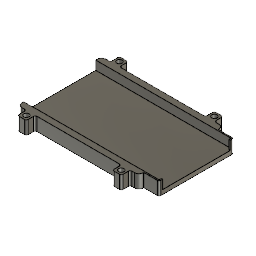
Assembled_v1 (Autodesk Fusion 360 archive; units mm, degrees)
design "fan_bottom_96"
Autodesk Fusion 360 part; units mm, degrees
(part 1 of 2)
sketch "Sketch1" plane through (0, 0, 0) normal (0, 0, 1) x (1, 0, 0)
  line L0 (-68.38, 47.37) -> (68.38, 47.37)
  line L1 (68.38, 47.37) -> (68.38, -47.37)
  line L2 (68.38, -47.37) -> (-68.38, -47.37)
  line L3 (-68.38, -47.37) -> (-68.38, 47.37)
  line L4 (-68.38, 47.37) -> (68.38, -47.37) construction
  line L5 (68.38, 47.37) -> (-68.38, -47.37) construction
  line L6 (-58.38, 57.37) -> (-48.38, 57.37)
  line L7 (-48.38, 57.37) -> (-48.38, 47.37)
  line L8 (-48.38, 47.37) -> (-58.38, 47.37)
  line L9 (-58.38, 47.37) -> (-58.38, 57.37)
  line L10 (48.38, 57.37) -> (58.38, 57.37)
  line L11 (58.38, 57.37) -> (58.38, 47.37)
  line L12 (58.38, 47.37) -> (48.38, 47.37)
  line L13 (48.38, 47.37) -> (48.38, 57.37)
  line L14 (48.38, -47.37) -> (58.38, -47.37)
  line L15 (58.38, -47.37) -> (58.38, -57.37)
  line L16 (58.38, -57.37) -> (48.38, -57.37)
  line L17 (48.38, -57.37) -> (48.38, -47.37)
  line L18 (-58.38, -47.37) -> (-48.38, -47.37)
  line L19 (-48.38, -47.37) -> (-48.38, -57.37)
  line L20 (-48.38, -57.37) -> (-58.38, -57.37)
  line L21 (-58.38, -57.37) -> (-58.38, -47.37)
  point P0 (-57.3369, -42.2056)
  point P1 (-53.88, -84.89)
  dimension "d1" = 136.76
  dimension "d2" = 94.74
  dimension "d3" = 10
  dimension "d4" = 10
  dimension "d5" = 10
  dimension "d6" = 10
  constraint perpendicular L0 L1
  constraint parallel L0 L2
  constraint parallel L1 L3
  constraint horizontal L0
  constraint horizontal L6
  constraint vertical L7
  constraint horizontal L8
  constraint vertical L9
  constraint coincident L0 L7.end
  constraint horizontal L10
  constraint vertical L11
  constraint horizontal L12
  constraint vertical L13
  constraint horizontal L14
  constraint vertical L15
  constraint horizontal L16
  constraint vertical L17
  constraint horizontal L18
  constraint vertical L19
  constraint horizontal L20
  constraint vertical L21
  measures "d1" distance of L1 L3
  measures "d2" distance of L0.start L2.end
  measures "d3" distance of L6.start L6.end
  measures "d4" distance of L6.start L8.end
  measures "d5" distance of L10.start L10.end
  measures "d6" distance of L10.start L12.end
extrude "Extrude1" add sketch "Sketch1" along normal blind 15
ref_plane "WorkPlane1" through (0, 0, 15) normal (0, 0, 1) x (1, 0, 0)
sketch "Sketch2" plane through (0, 0, 15) normal (0, 0, 1) x (1, 0, 0)
  line L0 (68.38, -40.5) -> (-68.38, -40.5)
  line L1 (-68.38, -40.5) -> (-68.38, 40.5)
  line L2 (-68.38, 40.5) -> (68.38, 40.5)
  line L3 (68.38, 40.5) -> (68.38, -40.5)
  line L4 (68.38, -40.5) -> (-68.38, 40.5) construction
  line L5 (-68.38, -40.5) -> (68.38, 40.5) construction
  dimension "d18" = 136.76
  dimension "d19" = 81
  constraint perpendicular L0 L1
  constraint parallel L0 L2
  constraint parallel L1 L3
  constraint horizontal L0
  constraint coincident L4 origin
  constraint coincident L5 origin
  measures "d18" distance of L1.end L2.end
  measures "d19" distance of L0.end L1.end
extrude "Extrude2" cut sketch "Sketch2" against normal blind 10
ref_plane "WorkPlane2" through (68.38, 0, 7.5) normal (1, 0, 0) x (0, 1, 0)
sketch "Sketch3" plane through (68.38, 0, 7.5) normal (1, 0, 0) x (0, 1, 0)
  line L0 (42, -7.5) -> (-42, -7.5)
  line L1 (-42, -7.5) -> (-42, 7.5)
  line L2 (-42, 7.5) -> (42, 7.5)
  line L3 (42, 7.5) -> (42, -7.5)
  line L4 (42, -7.5) -> (-42, 7.5) construction
  line L5 (-42, -7.5) -> (42, 7.5) construction
  dimension "d23" = 84
  dimension "d24" = 15
  constraint perpendicular L0 L1
  constraint parallel L0 L2
  constraint parallel L1 L3
  constraint horizontal L0
  constraint coincident L4 origin
  constraint coincident L5 origin
  measures "d23" distance of L1.end L2.end
  measures "d24" distance of L0.end L1.end
sketch "Sketch5" plane through (7.88, 0, 15) normal (0, 0, 1) x (1, 0, 0)
  circle A0 centre (-61.26, 52.37) radius 3
  circle A1 centre (45.5, 52.37) radius 3
  circle A2 centre (-61.26, -52.37) radius 3
  circle A3 centre (45.5, -52.37) radius 3
  dimension "d29" = 6
  dimension "d32" = 106.76
  dimension "d33" = -104.74
  measures "d29" diameter of A0
extrude "Extrude4" cut sketch "Sketch5" against normal blind 15
fillet "Fillet4" radius 5 4 edges at (68.38, 47.37, 7.5) (-68.38, 47.37, 7.5) (-68.38, -47.37, 7.5) (68.38, -47.37, 7.5)
ref_plane "WorkPlane7" through (68.38, 0, 7.5) normal (1, 0, 0) x (0, 1, 0)
fillet "Fillet5" radius 2 16 edges at (-58.38, -57.37, 7.5) (-48.38, -57.37, 7.5) (-48.38, -47.37, 7.5) (48.38, -57.37, 7.5) (58.38, -57.37, 7.5) (58.38, -47.37, 7.5) (58.38, 47.37, 7.5) (58.38, 57.37, 7.5) (48.38, 57.37, 7.5) (-48.38, 47.37, 7.5) (-48.38, 57.37, 7.5) (-58.38, 57.37, 7.5) (48.38, 47.37, 7.5) (-58.38, 47.37, 7.5) (-58.38, -47.37, 7.5) (48.38, -47.37, 7.5)
sketch "Sketch8" plane through (68.38, 0, 7.5) normal (1, 0, 0) x (0, 1, 0)
  line L0 (0, -7.5) -> (-42, -7.5)
  line L1 (-42, -7.5) -> (42, -7.5)
  line L2 (42, -7.5) -> (42, 7.5)
  line L3 (42, 7.5) -> (-42, 7.5)
  line L4 (-42, 7.5) -> (-42, -7.5)
  dimension "d52" = 42
  dimension "d53" = 84
  dimension "d54" = 15
  constraint horizontal L0
  constraint horizontal L1
  constraint vertical L2
  constraint horizontal L3
  constraint vertical L4
  measures "d52" distance of L0.start L0.end
  measures "d53" distance of L0.end L1.end
  measures "d54" distance of L0.end L3.end
extrude "Extrude6" add sketch "Sketch8" along normal blind 17.2
ref_plane "WorkPlane9" through (8.6, 0, 15) normal (0, 0, 1) x (1, 0, 0)
sketch "Sketch10" plane through (8.6, 0, 15) normal (0, 0, 1) x (1, 0, 0)
  line L0 (75.48, -40.5) -> (44.08, -40.5)
  line L1 (44.08, -40.5) -> (44.08, 40.5)
  line L2 (44.08, 40.5) -> (75.48, 40.5)
  line L3 (75.48, 40.5) -> (75.48, -40.5)
  line L4 (75.48, -40.5) -> (44.08, 40.5) construction
  line L5 (44.08, -40.5) -> (75.48, 40.5) construction
  point P0 (59.78, 0)
  dimension "d66" = 31.4
  dimension "d67" = 81
  constraint perpendicular L0 L1
  constraint parallel L0 L2
  constraint parallel L1 L3
  constraint horizontal L0
  constraint coincident L4 P0
  constraint coincident L5 P0
  measures "d66" distance of L1.end L2.end
  measures "d67" distance of L0.end L1.end
extrude "Extrude8" cut sketch "Sketch10" against normal blind 10
fillet "Fillet8" radius 2 2 edges at (85.58, 42, 7.5) (85.58, -42, 7.5)
ref_plane "WorkPlane11" through (85.58, 0, 7.5) normal (1, 0, 0) x (0, 0, -1)
sketch "Sketch12" plane through (85.58, 0, 7.5) normal (1, 0, 0) x (0, 1, 0)
  line L0 (38, -2.5) -> (-38, -2.5)
  line L1 (-38, -2.5) -> (-38, 17.5)
  line L2 (-38, 17.5) -> (38, 17.5)
  line L3 (38, 17.5) -> (38, -2.5)
  line L4 (38, -2.5) -> (-38, 17.5) construction
  line L5 (-38, -2.5) -> (38, 17.5) construction
  point P0 (0, 7.5)
  dimension "d73" = 76
  dimension "d74" = 20
  constraint perpendicular L0 L1
  constraint parallel L0 L2
  constraint parallel L1 L3
  constraint horizontal L0
  constraint coincident L4 P0
  constraint coincident L5 P0
  measures "d73" distance of L1.end L2.end
  measures "d74" distance of L0.end L1.end
extrude "Extrude9" cut sketch "Sketch12" against normal blind 1.5

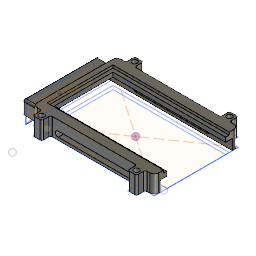
design "Mounting_plate_96_v2"
Autodesk Fusion 360 part; units mm, degrees
sketch "Sketch1" plane through (0, 0, 0) normal (0, 0, 1) x (1, 0, 0)
  line L0 (-68.38, 47.37) -> (68.38, 47.37)
  line L1 (68.38, 47.37) -> (68.38, -47.37)
  line L2 (68.38, -47.37) -> (-68.38, -47.37)
  line L3 (-68.38, -47.37) -> (-68.38, 47.37)
  line L4 (-68.38, 47.37) -> (68.38, -47.37) construction
  line L5 (68.38, 47.37) -> (-68.38, -47.37) construction
  line L6 (-58.38, 57.37) -> (-48.38, 57.37)
  line L7 (-48.38, 57.37) -> (-48.38, 47.37)
  line L8 (-48.38, 47.37) -> (-58.38, 47.37)
  line L9 (-58.38, 47.37) -> (-58.38, 57.37)
  line L10 (48.38, 57.37) -> (58.38, 57.37)
  line L11 (58.38, 57.37) -> (58.38, 47.37)
  line L12 (58.38, 47.37) -> (48.38, 47.37)
  line L13 (48.38, 47.37) -> (48.38, 57.37)
  line L14 (48.38, -47.37) -> (58.38, -47.37)
  line L15 (58.38, -47.37) -> (58.38, -57.37)
  line L16 (58.38, -57.37) -> (48.38, -57.37)
  line L17 (48.38, -57.37) -> (48.38, -47.37)
  line L18 (-58.38, -47.37) -> (-48.38, -47.37)
  line L19 (-48.38, -47.37) -> (-48.38, -57.37)
  line L20 (-48.38, -57.37) -> (-58.38, -57.37)
  line L21 (-58.38, -57.37) -> (-58.38, -47.37)
  line L22 (68.38, 47.37) -> (68.38, 37)
  line L23 (68.38, -47.37) -> (68.38, -36.63)
  line L24 (68.38, 37) -> (-62.58, 37)
  line L25 (-62.58, 37) -> (-62.58, -37)
  line L26 (-62.58, -37) -> (68.38, -37)
  line L27 (68.38, -37) -> (68.38, 37)
  line L28 (68.38, 37) -> (68.38, 33)
  line L29 (68.38, 33) -> (-58.58, 33)
  line L30 (-58.58, 33) -> (-58.58, -33)
  line L31 (-58.58, -33) -> (68.38, -33)
  line L32 (68.38, -33) -> (68.38, 33)
  point P0 (-57.3369, -42.2056)
  point P1 (-53.88, -84.89)
  dimension "d1" = 136.76
  dimension "d2" = 94.74
  dimension "d3" = 10
  dimension "d4" = 10
  dimension "d5" = 10
  dimension "d6" = 10
  dimension "d15" = 10.37
  dimension "d16" = 10.74
  dimension "d17" = 74
  dimension "d18" = 130.96
  dimension "d19" = 4
  dimension "d20" = 66
  dimension "d21" = 126.96
  constraint perpendicular L0 L1
  constraint parallel L0 L2
  constraint parallel L1 L3
  constraint horizontal L0
  constraint horizontal L6
  constraint vertical L7
  constraint horizontal L8
  constraint vertical L9
  constraint coincident L0 L7.end
  constraint horizontal L10
  constraint vertical L11
  constraint horizontal L12
  constraint vertical L13
  constraint horizontal L14
  constraint vertical L15
  constraint horizontal L16
  constraint vertical L17
  constraint horizontal L18
  constraint vertical L19
  constraint horizontal L20
  constraint vertical L21
  constraint perpendicular L0 L22
  constraint perpendicular L2 L23
  constraint horizontal L24
  constraint vertical L25
  constraint horizontal L26
  constraint vertical L27
  constraint perpendicular L24 L28
  constraint horizontal L29
  constraint vertical L30
  constraint horizontal L31
  constraint vertical L32
  measures "d1" distance of L1 L3
  measures "d2" distance of L0.start L2.end
  measures "d3" distance of L6.start L6.end
  measures "d4" distance of L6.start L8.end
  measures "d5" distance of L10.start L10.end
  measures "d6" distance of L10.start L12.end
  measures "d15" distance of L0.end L22.end
  measures "d16" distance of L1.end L23.end
  measures "d17" distance of L22.end L26.end
  measures "d18" distance of L22.end L24.end
  measures "d19" distance of L22.end L28.end
  measures "d20" distance of L28.end L31.end
  measures "d21" distance of L28.end L29.end
extrude "Extrude2" add sketch "Sketch1" along normal blind 20 contours L0 L1 L2 L3 L8 L12 L14 L18 L22 L23 L24 L25 L26 | L0 L6 L7 L8 L9 | L2 L18 L19 L20 L21 | L0 L10 L11 L12 L13 | L2 L14 L15 L16 L17 | L1 L23 L24 L25 L26 L27 L28 L29 L30 L31 makes body 1
ref_plane "WorkPlane2" through (0, 0, 20) normal (0, 0, 1) x (1, 0, 0)
sketch "Sketch4" plane through (0, 0, 20) normal (0, 0, 1) x (1, 0, 0)
  line L0 (68.38, 37) -> (-62.58, 37)
  line L1 (-62.58, 37) -> (-62.58, -37)
  line L2 (-62.58, -37) -> (68.38, -37)
  line L3 (68.38, -37) -> (68.38, 37)
  dimension "d30" = 130.96
  dimension "d31" = 74
  constraint horizontal L0
  constraint vertical L1
  constraint horizontal L2
  constraint vertical L3
  measures "d30" distance of L0.start L0.end
  measures "d31" distance of L0.start L2.end
extrude "Extrude3" cut sketch "Sketch4" against normal blind 3 bodies 1
ref_plane "WorkPlane3" through (0, 0, 20) normal (0, 0, 1) x (1, 0, 0)
sketch "Sketch5" plane through (0, 0, 20) normal (0, 0, 1) x (1, 0, 0)
  circle A0 centre (-53.38, 52.37) radius 3
  circle A1 centre (53.38, 52.37) radius 3
  circle A2 centre (-53.38, -52.37) radius 3
  circle A3 centre (53.38, -52.37) radius 3
  dimension "d35" = 6
  dimension "d38" = 106.76
  dimension "d39" = -104.74
  measures "d35" diameter of A0
extrude "Extrude4" cut sketch "Sketch5" against normal blind 20 bodies 1
ref_plane "WorkPlane5" through (68.38, 0, 0) normal (1, 0, 0) x (0, 1, 0)
ref_plane "WorkPlane6" through (68.38, 0, 0) normal (1, 0, 0) x (0, 1, 0)
sketch "Sketch7" plane through (68.38, 0, 0) normal (1, 0, 0) x (0, 1, 0)
  line L0 (40.5, 12) -> (-40.5, 12)
  line L1 (-40.5, 12) -> (-40.5, -12)
  line L2 (-40.5, -12) -> (40.5, -12)
  line L3 (40.5, -12) -> (40.5, 12)
  line L4 (40.5, 12) -> (-40.5, -12) construction
  line L5 (-40.5, 12) -> (40.5, -12) construction
  dimension "d45" = 81
  dimension "d46" = 24
  constraint perpendicular L0 L1
  constraint parallel L0 L2
  constraint parallel L1 L3
  constraint horizontal L0
  constraint coincident L4 origin
  constraint coincident L5 origin
  measures "d45" distance of L1.end L2.end
  measures "d46" distance of L0.end L1.end
extrude "Extrude5" cut sketch "Sketch7" against normal blind 136.76 bodies 1
fillet "Fillet1" radius 5 4 edges at (68.38, 47.37, 10) (-68.38, 47.37, 10) (-68.38, -47.37, 10) (68.38, -47.37, 10) on bodies 1
fillet "Fillet2" radius 2 16 edges at (-58.38, 57.37, 10) (-58.38, 47.37, 10) (-58.38, -47.37, 10) (-58.38, -57.37, 10) (-48.38, -57.37, 10) (-48.38, -47.37, 10) (58.38, -57.37, 10) (58.38, -47.37, 10) (48.38, -47.37, 10) (48.38, -57.37, 10) (58.38, 47.37, 10) (58.38, 57.37, 10) (48.38, 47.37, 10) (48.38, 57.37, 10) (-48.38, 47.37, 10) (-48.38, 57.37, 10) on bodies 1
ref_plane "WorkPlane7" through (0, -47.37, 10) normal (0, -1, 0) x (1, 0, 0)
delete_face "DeleteFace1" 1 faces at (15.46, -47.37, 6.6667) on bodies 1
ref_plane "WorkPlane9" through (0, -47.37, 10) normal (0, -1, 0) x (1, 0, 0)
sketch "Sketch10" plane through (0, -47.37, 10) normal (0, -1, 0) x (1, 0, 0)
  line L0 (0, -10) -> (0, -4)
  line L1 (40, -7) -> (-40, -7)
  line L2 (-40, -7) -> (-40, -1)
  line L3 (-40, -1) -> (40, -1)
  line L4 (40, -1) -> (40, -7)
  line L5 (40, -7) -> (-40, -1) construction
  line L6 (-40, -7) -> (40, -1) construction
  circle A0 centre (-40, -4) radius 3
  circle A1 centre (40, -4) radius 3
  point P0 (0, -4)
  dimension "d72" = 6
  dimension "d73" = 6
  dimension "d74" = 80
  dimension "d75" = 6
  dimension "d76" = 6
  constraint vertical L0
  constraint perpendicular L1 L2
  constraint parallel L1 L3
  constraint parallel L2 L4
  constraint horizontal L1
  constraint coincident L5 P0
  constraint coincident L6 P0
  constraint coincident P0 L0.end
  constraint midpoint L2 A0.centre
  constraint midpoint L4 A1.centre
  measures "d72" distance of L0.start P0
  measures "d73" distance of L1.end L2.end
  measures "d74" distance of L2.end L3.end
  measures "d75" diameter of A0
  measures "d76" diameter of A1
extrude "Extrude9" cut sketch "Sketch10" against normal blind 6.87 bodies 1
ref_plane "WorkPlane10" through (0, 47.37, 10) normal (0, 1, 0) x (-1, 0, 0)
sketch "Sketch11" plane through (0, 47.37, 10) normal (0, 1, 0) x (1, 0, 0)
  line L0 (0, 10) -> (0, 4)
  line L1 (-40, 7) -> (40, 7)
  line L2 (40, 7) -> (40, 1)
  line L3 (40, 1) -> (-40, 1)
  line L4 (-40, 1) -> (-40, 7)
  line L5 (-40, 7) -> (40, 1) construction
  line L6 (40, 7) -> (-40, 1) construction
  circle A0 centre (40, 4) radius 3
  circle A1 centre (-40, 4) radius 3
  point P0 (0, 4)
  dimension "d80" = 6
  dimension "d81" = 80
  dimension "d82" = 6
  dimension "d83" = 6
  dimension "d84" = 6
  constraint vertical L0
  constraint perpendicular L1 L2
  constraint parallel L1 L3
  constraint parallel L2 L4
  constraint horizontal L1
  constraint coincident L5 P0
  constraint coincident L6 P0
  constraint coincident P0 L0.end
  constraint midpoint L2 A0.centre
  constraint midpoint L4 A1.centre
  measures "d80" distance of L0.start P0
  measures "d81" distance of L2.end L3.end
  measures "d82" distance of L1.end L2.end
  measures "d83" diameter of A0
  measures "d84" diameter of A1
extrude "Extrude10" cut sketch "Sketch11" against normal blind 6.87 bodies 1
ref_plane "WorkPlane11" through (0, 0, 0) normal (0, 0, 1) x (1, 0, 0)
sketch "Sketch12" plane through (0, 0, 0) normal (0, 0, 1) x (1, 0, 0)
ref_plane "WorkPlane12" through (-68.38, 0, 10) normal (-1, 0, 0) x (0, -1, 0)
ref_plane "WorkPlane13" through (-68.38, 0, 10) normal (-1, 0, 0) x (0, -1, 0)
sketch "Sketch19" plane through (68.38, 0, 0) normal (1, 0, 0) x (0, 1, 0)
ref_plane "WorkPlane19" through (-68.38, 0, 10) normal (-1, 0, 0) x (0, -1, 0)
sketch "Sketch21" plane through (-68.38, 0, 10) normal (-1, 0, 0) x (0, 1, 0)
  line L0 (42, -2) -> (-42, -2)
  line L1 (42, -2) -> (-42, 22) construction
  line L2 (-42, -2) -> (42, 22) construction
  line L3 (42, -2) -> (-42, -2)
  line L4 (-42, -2) -> (-42, 10)
  line L5 (-42, 10) -> (42, 10)
  line L6 (42, 10) -> (42, -2)
  point P0 (0, 10)
  dimension "d112" = 84
  dimension "d113" = 24
  constraint horizontal L0
  constraint coincident L1 P0
  constraint coincident L2 P0
  constraint horizontal L3
  constraint vertical L4
  constraint horizontal L5
  constraint vertical L6
  measures "d112" distance of L1.end L2.end
  measures "d113" distance of L0.end L1.end
extrude "Extrude15" add sketch "Sketch21" along normal blind 17.2 separate body makes body 2
ref_plane "WorkPlane20" through (-68.32, 0, 0) normal (1, 0, 0) x (0, 1, 0)
sketch "Sketch22" plane through (-68.32, 0, 0) normal (1, 0, 0) x (0, 1, 0)
  line L0 (40.5, -12) -> (-40.5, -12)
  line L1 (-40.5, -12) -> (-40.5, 12)
  line L2 (-40.5, 12) -> (40.5, 12)
  line L3 (40.5, 12) -> (40.5, -12)
  line L4 (40.5, -12) -> (-40.5, 12) construction
  line L5 (-40.5, -12) -> (40.5, 12) construction
  dimension "d117" = 81
  dimension "d118" = 24
  constraint perpendicular L0 L1
  constraint parallel L0 L2
  constraint parallel L1 L3
  constraint horizontal L0
  constraint coincident L4 origin
  constraint coincident L5 origin
  measures "d117" distance of L1.end L2.end
  measures "d118" distance of L0.end L1.end
extrude "Extrude16" cut sketch "Sketch22" against normal blind 15.76 bodies 2
ref_plane "WorkPlane23" through (-76.98, 0, 12) normal (0, 0, 1) x (0, 1, 0)
sketch "Sketch25" plane through (-76.98, 0, 12) normal (0, 0, 1) x (1, 0, 0)
  line L0 (8.6, 42) -> (-8.6, 42)
  line L1 (-8.6, 42) -> (-8.6, -42)
  line L2 (-8.6, -42) -> (8.6, -42)
  line L3 (8.6, -42) -> (8.6, 42)
  dimension "d136" = 17.2
  dimension "d137" = 84
  constraint horizontal L0
  constraint vertical L1
  constraint horizontal L2
  constraint vertical L3
  measures "d136" distance of L0.start L0.end
  measures "d137" distance of L0.start L2.end
extrude "Extrude19" add sketch "Sketch25" along normal blind 3 bodies 1 2
fillet "Fillet5" radius 2 5 edges at (-76.98, 42, 15) (-85.58, 42, 7.5) (-85.58, 0, 15) (-76.98, -42, 15) (-85.58, -42, 7.5) on bodies 1
ref_plane "WorkPlane24" through (-85.58, 0, 6.5) normal (-1, 0, 0) x (0, -1, 0)
sketch "Sketch26" plane through (-85.58, 0, 6.5) normal (-1, 0, 0) x (0, 1, 0)
  line L0 (38, 18.5) -> (-38, 18.5)
  line L1 (-38, 18.5) -> (-38, -3.5)
  line L2 (-38, -3.5) -> (38, -3.5)
  line L3 (38, -3.5) -> (38, 18.5)
  line L4 (38, 18.5) -> (-38, -3.5) construction
  line L5 (-38, 18.5) -> (38, -3.5) construction
  point P0 (0, 7.5)
  dimension "d142" = 76
  dimension "d143" = 22
  constraint perpendicular L0 L1
  constraint parallel L0 L2
  constraint parallel L1 L3
  constraint horizontal L0
  constraint coincident L4 P0
  constraint coincident L5 P0
  measures "d142" distance of L1.end L2.end
  measures "d143" distance of L0.end L1.end
extrude "Extrude21" cut sketch "Sketch26" against normal blind 17.2 bodies 1
extrude "Extrude20" [rolled back] along distance -17.2 taper angle 0
fillet "Fillet3" [rolled back] radius 2
fillet "Fillet4" [rolled back] radius 2
ref_plane "WorkPlane21" through (-85.58, 0, 5) normal (-1, 0, 0) x (0, 0, 1)
ref_plane "WorkPlane22" through (-85.58, 0, 5) normal (-1, 0, 0) x (0, 0, 1)
sketch "Sketch24" plane through (-85.58, 0, 5) normal (-1, 0, 0) x (0, 1, 0)
  line L0 (-38, 11) -> (38, 11)
  line L1 (38, 11) -> (38, -3)
  line L2 (38, -3) -> (-38, -3)
  line L3 (-38, -3) -> (-38, 11)
  line L4 (-38, 11) -> (38, -3) construction
  line L5 (38, 11) -> (-38, -3) construction
  point P0 (0, 4)
  dimension "d131" = 76
  dimension "d132" = 14
  constraint perpendicular L0 L1
  constraint parallel L0 L2
  constraint parallel L1 L3
  constraint horizontal L0
  constraint coincident L4 P0
  constraint coincident L5 P0
  measures "d131" distance of L1.end L2.end
  measures "d132" distance of L0.end L1.end
extrude "Extrude18" [rolled back] along distance -1.5 taper angle 0

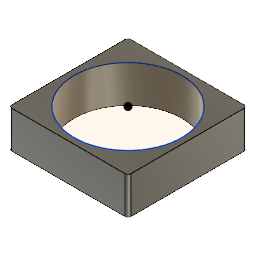
design "Fan"
Autodesk Fusion 360 part; units mm, degrees
sketch "Sketch1" plane through (0, 0, 0) normal (0, 0, 1) x (1, 0, 0)
  line L0 (40, -40) -> (-40, -40)
  line L1 (-40, -40) -> (-40, 40)
  line L2 (-40, 40) -> (40, 40)
  line L3 (40, 40) -> (40, -40)
  line L4 (40, -40) -> (-40, 40) construction
  line L5 (-40, -40) -> (40, 40) construction
  dimension "d1" = 80
  dimension "d2" = 80
  constraint perpendicular L0 L1
  constraint parallel L0 L2
  constraint parallel L1 L3
  constraint horizontal L0
  constraint coincident L4 origin
  constraint coincident L5 origin
  measures "d1" distance of L1.end L2.end
  measures "d2" distance of L0.end L1.end
extrude "Extrude1" add sketch "Sketch1" along normal blind 25
ref_plane "WorkPlane1" through (0, 0, 25) normal (0, 0, 1) x (1, 0, 0)
sketch "Sketch2" plane through (0, 0, 25) normal (0, 0, 1) x (1, 0, 0)
  circle A0 centre (0, 0) radius 36.0555
  constraint coincident A0.centre origin
extrude "Extrude3" cut sketch "Sketch2" against normal blind 25
fillet "Fillet1" radius 2 4 edges at (40, -40, 12.5) (40, 40, 12.5) (-40, 40, 12.5) (-40, -40, 12.5)

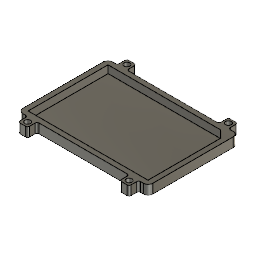
design "plate_lid_sketch"
Autodesk Fusion 360 part; units mm, degrees
sketch "Sketch1" plane through (0, 0, 0) normal (0, 0, 1) x (1, 0, 0)
  line L0 (68.38, -47.235) -> (-68.38, -47.235)
  line L1 (-68.38, -47.235) -> (-68.38, 47.235)
  line L2 (-68.38, 47.235) -> (68.38, 47.235)
  line L3 (68.38, 47.235) -> (68.38, -47.235)
  line L4 (68.38, -47.235) -> (-68.38, 47.235) construction
  line L5 (-68.38, -47.235) -> (68.38, 47.235) construction
  line L6 (-48.38, 47.235) -> (-58.38, 47.235)
  line L7 (-58.38, 47.235) -> (-58.38, 57.235)
  line L8 (-58.38, 57.235) -> (-48.38, 57.235)
  line L9 (-48.38, 57.235) -> (-48.38, 47.235)
  line L10 (-48.38, 47.235) -> (-58.38, 57.235) construction
  line L11 (-58.38, 47.235) -> (-48.38, 57.235) construction
  line L12 (48.38, 57.235) -> (58.38, 57.235)
  line L13 (48.38, 47.235) -> (48.38, 57.235)
  line L14 (58.38, 57.235) -> (58.38, 47.235)
  line L15 (58.38, 47.235) -> (48.38, 47.235)
  line L16 (48.38, -57.235) -> (48.38, -47.235)
  line L17 (48.38, -47.235) -> (58.38, -47.235)
  line L18 (58.38, -47.235) -> (58.38, -57.235)
  line L19 (48.38, -57.235) -> (58.38, -57.235)
  line L20 (-58.38, -57.235) -> (-58.38, -47.235)
  line L21 (-58.38, -47.235) -> (-48.38, -47.235)
  line L22 (-48.38, -47.235) -> (-48.38, -57.235)
  line L23 (-48.38, -57.235) -> (-58.38, -57.235)
  point P0 (-53.38, 52.235)
  dimension "d1" = 136.76
  dimension "d2" = 94.47
  dimension "d3" = 10
  dimension "d4" = 10
  dimension "d6" = 10
  dimension "d7" = 10
  constraint perpendicular L0 L1
  constraint parallel L0 L2
  constraint parallel L1 L3
  constraint horizontal L0
  constraint coincident L4 origin
  constraint coincident L5 origin
  constraint perpendicular L6 L7
  constraint parallel L6 L8
  constraint parallel L7 L9
  constraint horizontal L6
  constraint coincident L10 P0
  constraint coincident L11 P0
  constraint perpendicular L13 L15
  constraint parallel L12 L15
  constraint parallel L13 L14
  constraint horizontal L15
  constraint parallel L16 L18
  constraint perpendicular L18 L19
  constraint perpendicular L20 L23
  constraint parallel L21 L23
  constraint parallel L20 L22
  constraint horizontal L23
  measures "d1" distance of L1.end L2.end
  measures "d2" distance of L0.end L1.end
  measures "d3" distance of L6.end L7.end
  measures "d4" distance of L13.start L12.start
  measures "d6" distance of L16.start L16.end
  measures "d7" distance of L20.start L20.end
extrude "Extrude1" add sketch "Sketch1" along normal blind 10 and the other way blind 0
ref_plane "WorkPlane1" through (0, 0, 10) normal (0, 0, 1) x (1, 0, 0)
sketch "Sketch2" plane through (0, 0, 10) normal (0, 0, 1) x (1, 0, 0)
  line L0 (62.5, -41.5) -> (-62.5, -41.5)
  line L1 (-62.5, -41.5) -> (-62.5, 41.5)
  line L2 (-62.5, 41.5) -> (62.5, 41.5)
  line L3 (62.5, 41.5) -> (62.5, -41.5)
  line L4 (62.5, -41.5) -> (-62.5, 41.5) construction
  line L5 (-62.5, -41.5) -> (62.5, 41.5) construction
  line L6 (-62.5, -41.5) -> (-62.5, 34.9)
  line L7 (62.5, 41.5) -> (-55.8, 41.5)
  line L8 (-62.5, 34.9) -> (-55.8, 41.5)
  dimension "d13" = 125
  dimension "d14" = 83
  dimension "d15" = 76.4
  dimension "d16" = 118.3
  constraint perpendicular L0 L1
  constraint parallel L0 L2
  constraint parallel L1 L3
  constraint horizontal L0
  constraint coincident L4 origin
  constraint coincident L5 origin
  constraint perpendicular L0 L6
  constraint perpendicular L3 L7
  measures "d13" distance of L1.end L2.end
  measures "d14" distance of L0.end L1.end
  measures "d15" distance of L0.end L6.end
  measures "d16" distance of L2.end L7.end
extrude "Extrude2" cut sketch "Sketch2" against normal blind 8 contours L0 L1 L2 L3 L6 L7 L8
ref_plane "WorkPlane2" through (0, 0, 10) normal (0, 0, 1) x (1, 0, 0)
sketch "Sketch3" plane through (0, 0, 10) normal (0, 0, 1) x (1, 0, 0)
  circle A0 centre (-53.3802, 52.2353) radius 3
  circle A1 centre (53.38, 52.2349) radius 3
  circle A2 centre (53.3799, -52.2347) radius 3
  circle A3 centre (-53.3802, -52.2349) radius 3
  dimension "d20" = 6
  dimension "d21" = 6
  dimension "d22" = 6
  dimension "d23" = 6
  measures "d20" diameter of A0
  measures "d21" diameter of A1
  measures "d22" diameter of A2
  measures "d23" diameter of A3
extrude "Extrude3" cut sketch "Sketch3" against normal blind 10
fillet "Fillet1" radius 5 4 edges at (68.38, -47.235, 5) (68.38, 47.235, 5) (-68.38, -47.235, 5) (-68.38, 47.235, 5)
fillet "Fillet2" radius 2 16 edges at (58.38, -47.235, 5) (58.38, -57.235, 5) (48.38, -57.235, 5) (58.38, 57.235, 5) (-48.38, -47.235, 5) (-48.38, -57.235, 5) (-58.38, -57.235, 5) (-48.38, 57.235, 5) (58.38, 47.235, 5) (-48.38, 47.235, 5) (-58.38, 57.235, 5) (48.38, 57.235, 5) (48.38, 47.235, 5) (-58.38, 47.235, 5) (48.38, -47.235, 5) (-58.38, -47.235, 5)
extrude "Extrude4" add 1 faces at (-18.6, -13.8333, 2) along direction (0, 0, 1) blind 8
ref_plane "WorkPlane3" through (0, 0, 10) normal (0, 0, 1) x (1, 0, 0)
sketch "Sketch4" plane through (0, 0, 10) normal (0, 0, 1) x (1, 0, 0)
  line L0 (63, -42) -> (-63, -42)
  line L1 (-63, -42) -> (-63, 42)
  line L2 (-63, 42) -> (63, 42)
  line L3 (63, 42) -> (63, -42)
  line L4 (63, -42) -> (-63, 42) construction
  line L5 (-63, -42) -> (63, 42) construction
  line L6 (63, -42) -> (63, 34.4)
  line L7 (-63, 42) -> (55.3, 42)
  line L8 (55.3, 42) -> (63, 34.4)
  dimension "d31" = 126
  dimension "d32" = 84
  dimension "d33" = 76.4
  dimension "d34" = 118.3
  constraint perpendicular L0 L1
  constraint parallel L0 L2
  constraint parallel L1 L3
  constraint horizontal L0
  constraint coincident L4 origin
  constraint coincident L5 origin
  constraint perpendicular L0 L6
  constraint perpendicular L1 L7
  measures "d31" distance of L1.end L2.end
  measures "d32" distance of L0.end L1.end
  measures "d33" distance of L0.start L6.end
  measures "d34" distance of L1.end L7.end
extrude "Extrude6" cut sketch "Sketch4" against normal blind 8 contours L0 L1 L2 L3 L6 L7 L8
extrude "Extrude5" cut sketch "Sketch4" against normal blind 8 contours L0 L1 L2 L3 L6 L7 L8

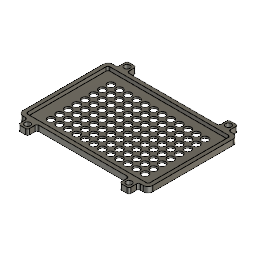
design "Plate_Adapter_96_4mm_thickness"
Autodesk Fusion 360 part; units mm, degrees
sketch "Sketch1" plane through (0, 0, 0) normal (0, 0, 1) x (1, 0, 0)
  line L0 (-68.38, 47.37) -> (68.38, 47.37)
  line L1 (68.38, 47.37) -> (68.38, -47.37)
  line L2 (68.38, -47.37) -> (-68.38, -47.37)
  line L3 (-68.38, -47.37) -> (-68.38, 47.37)
  line L4 (-68.38, 47.37) -> (68.38, -47.37) construction
  line L5 (68.38, 47.37) -> (-68.38, -47.37) construction
  line L6 (-58.38, 57.37) -> (-48.38, 57.37)
  line L7 (-48.38, 57.37) -> (-48.38, 47.37)
  line L8 (-48.38, 47.37) -> (-58.38, 47.37)
  line L9 (-58.38, 47.37) -> (-58.38, 57.37)
  line L10 (48.38, 57.37) -> (58.38, 57.37)
  line L11 (58.38, 57.37) -> (58.38, 47.37)
  line L12 (58.38, 47.37) -> (48.38, 47.37)
  line L13 (48.38, 47.37) -> (48.38, 57.37)
  line L14 (48.38, -47.37) -> (58.38, -47.37)
  line L15 (58.38, -47.37) -> (58.38, -57.37)
  line L16 (58.38, -57.37) -> (48.38, -57.37)
  line L17 (48.38, -57.37) -> (48.38, -47.37)
  line L18 (-58.38, -47.37) -> (-48.38, -47.37)
  line L19 (-48.38, -47.37) -> (-48.38, -57.37)
  line L20 (-48.38, -57.37) -> (-58.38, -57.37)
  line L21 (-58.38, -57.37) -> (-58.38, -47.37)
  line L22 (-49.5, 31.5) -> (49.5, 31.5)
  line L23 (49.5, 31.5) -> (49.5, -31.5)
  line L24 (49.5, -31.5) -> (-49.5, -31.5)
  line L25 (-49.5, -31.5) -> (-49.5, 31.5)
  line L26 (-49.5, 31.5) -> (49.5, -31.5) construction
  line L27 (49.5, 31.5) -> (-49.5, -31.5) construction
  circle A0 centre (-49.5, -31.5) radius 3.575
  circle A1 centre (-40.5, -31.5) radius 3.575
  circle A2 centre (-31.5, -31.5) radius 3.575
  circle A3 centre (-22.5, -31.5) radius 3.575
  circle A4 centre (-13.5, -31.5) radius 3.575
  circle A5 centre (-4.5, -31.5) radius 3.575
  circle A6 centre (4.5, -31.5) radius 3.575
  circle A7 centre (13.5, -31.5) radius 3.575
  circle A8 centre (22.5, -31.5) radius 3.575
  circle A9 centre (31.5, -31.5) radius 3.575
  circle A10 centre (40.5, -31.5) radius 3.575
  circle A11 centre (49.5, -31.5) radius 3.575
  circle A12 centre (-49.5, -22.5) radius 3.575
  circle A13 centre (-40.5, -22.5) radius 3.575
  circle A14 centre (-31.5, -22.5) radius 3.575
  circle A15 centre (-22.5, -22.5) radius 3.575
  circle A16 centre (-13.5, -22.5) radius 3.575
  circle A17 centre (-4.5, -22.5) radius 3.575
  circle A18 centre (4.5, -22.5) radius 3.575
  circle A19 centre (13.5, -22.5) radius 3.575
  circle A20 centre (22.5, -22.5) radius 3.575
  circle A21 centre (31.5, -22.5) radius 3.575
  circle A22 centre (40.5, -22.5) radius 3.575
  circle A23 centre (49.5, -22.5) radius 3.575
  circle A24 centre (-49.5, -13.5) radius 3.575
  circle A25 centre (-40.5, -13.5) radius 3.575
  circle A26 centre (-31.5, -13.5) radius 3.575
  circle A27 centre (-22.5, -13.5) radius 3.575
  circle A28 centre (-13.5, -13.5) radius 3.575
  circle A29 centre (-4.5, -13.5) radius 3.575
  circle A30 centre (4.5, -13.5) radius 3.575
  circle A31 centre (13.5, -13.5) radius 3.575
  circle A32 centre (22.5, -13.5) radius 3.575
  circle A33 centre (31.5, -13.5) radius 3.575
  circle A34 centre (40.5, -13.5) radius 3.575
  circle A35 centre (49.5, -13.5) radius 3.575
  circle A36 centre (-49.5, -4.5) radius 3.575
  circle A37 centre (-40.5, -4.5) radius 3.575
  circle A38 centre (-31.5, -4.5) radius 3.575
  circle A39 centre (-22.5, -4.5) radius 3.575
  circle A40 centre (-13.5, -4.5) radius 3.575
  circle A41 centre (-4.5, -4.5) radius 3.575
  circle A42 centre (4.5, -4.5) radius 3.575
  circle A43 centre (13.5, -4.5) radius 3.575
  circle A44 centre (22.5, -4.5) radius 3.575
  circle A45 centre (31.5, -4.5) radius 3.575
  circle A46 centre (40.5, -4.5) radius 3.575
  circle A47 centre (49.5, -4.5) radius 3.575
  circle A48 centre (-49.5, 4.5) radius 3.575
  circle A49 centre (-40.5, 4.5) radius 3.575
  circle A50 centre (-31.5, 4.5) radius 3.575
  circle A51 centre (-22.5, 4.5) radius 3.575
  circle A52 centre (-13.5, 4.5) radius 3.575
  circle A53 centre (-4.5, 4.5) radius 3.575
  circle A54 centre (4.5, 4.5) radius 3.575
  circle A55 centre (13.5, 4.5) radius 3.575
  circle A56 centre (22.5, 4.5) radius 3.575
  circle A57 centre (31.5, 4.5) radius 3.575
  circle A58 centre (40.5, 4.5) radius 3.575
  circle A59 centre (49.5, 4.5) radius 3.575
  circle A60 centre (-49.5, 13.5) radius 3.575
  circle A61 centre (-40.5, 13.5) radius 3.575
  circle A62 centre (-31.5, 13.5) radius 3.575
  circle A63 centre (-22.5, 13.5) radius 3.575
  circle A64 centre (-13.5, 13.5) radius 3.575
  circle A65 centre (-4.5, 13.5) radius 3.575
  circle A66 centre (4.5, 13.5) radius 3.575
  circle A67 centre (13.5, 13.5) radius 3.575
  circle A68 centre (22.5, 13.5) radius 3.575
  circle A69 centre (31.5, 13.5) radius 3.575
  circle A70 centre (40.5, 13.5) radius 3.575
  circle A71 centre (49.5, 13.5) radius 3.575
  circle A72 centre (-49.5, 22.5) radius 3.575
  circle A73 centre (-40.5, 22.5) radius 3.575
  circle A74 centre (-31.5, 22.5) radius 3.575
  circle A75 centre (-22.5, 22.5) radius 3.575
  circle A76 centre (-13.5, 22.5) radius 3.575
  circle A77 centre (-4.5, 22.5) radius 3.575
  circle A78 centre (4.5, 22.5) radius 3.575
  circle A79 centre (13.5, 22.5) radius 3.575
  circle A80 centre (22.5, 22.5) radius 3.575
  circle A81 centre (31.5, 22.5) radius 3.575
  circle A82 centre (40.5, 22.5) radius 3.575
  circle A83 centre (49.5, 22.5) radius 3.575
  circle A84 centre (-49.5, 31.5) radius 3.575
  circle A85 centre (-40.5, 31.5) radius 3.575
  circle A86 centre (-31.5, 31.5) radius 3.575
  circle A87 centre (-22.5, 31.5) radius 3.575
  circle A88 centre (-13.5, 31.5) radius 3.575
  circle A89 centre (-4.5, 31.5) radius 3.575
  circle A90 centre (4.5, 31.5) radius 3.575
  circle A91 centre (13.5, 31.5) radius 3.575
  circle A92 centre (22.5, 31.5) radius 3.575
  circle A93 centre (31.5, 31.5) radius 3.575
  circle A94 centre (40.5, 31.5) radius 3.575
  circle A95 centre (49.5, 31.5) radius 3.575
  point P0 (-57.3369, -42.2056)
  point P1 (-53.88, -84.89)
  dimension "d1" = 136.76
  dimension "d2" = 94.74
  dimension "d3" = 10
  dimension "d4" = 10
  dimension "d5" = 10
  dimension "d6" = 10
  dimension "d7" = 63
  dimension "d8" = 99
  dimension "d10" = 7.15
  dimension "d13" = 99
  dimension "d14" = 63
  constraint perpendicular L0 L1
  constraint parallel L0 L2
  constraint parallel L1 L3
  constraint horizontal L0
  constraint coincident L4 origin
  constraint coincident L5 origin
  constraint horizontal L6
  constraint vertical L7
  constraint horizontal L8
  constraint vertical L9
  constraint coincident L0 L7.end
  constraint horizontal L10
  constraint vertical L11
  constraint horizontal L12
  constraint vertical L13
  constraint horizontal L14
  constraint vertical L15
  constraint horizontal L16
  constraint vertical L17
  constraint horizontal L18
  constraint vertical L19
  constraint horizontal L20
  constraint vertical L21
  constraint perpendicular L22 L23
  constraint parallel L22 L24
  constraint parallel L23 L25
  constraint horizontal L22
  constraint coincident L26 origin
  constraint coincident L27 origin
  measures "d1" distance of L1 L3
  measures "d2" distance of L0.start L2.end
  measures "d3" distance of L6.start L6.end
  measures "d4" distance of L6.start L8.end
  measures "d5" distance of L10.start L10.end
  measures "d6" distance of L10.start L12.end
  measures "d7" distance of L22.end L23.end
  measures "d8" distance of L23.end L24.end
  measures "d10" diameter of A0
extrude "Extrude1" add sketch "Sketch1" along normal mid plane 6 contours L0 L1 L2 L3 L8 L12 L14 L18 | L0 L6 L7 L8 L9 | L2 L18 L19 L20 L21 | L0 L10 L11 L12 L13 | L2 L14 L15 L16 L17 | L22 L23 L24 L25 A0 A1 A2 A3 A4 A5 A6 A7 A8 A9 A10 A11 A12 A23 A24 A35 A36 A47 A48 A59 A60 A71 A72 A83 A84 A85 A86 A87 A88 A89 A90 A91 A92 A93 A94 A95
ref_plane "WorkPlane1" through (0, 0, 3) normal (0, 0, 1) x (1, 0, 0)
sketch "Sketch2" plane through (0, 0, 3) normal (0, 0, 1) x (1, 0, 0)
  line L0 (-64.38, 43.235) -> (64.38, 43.235)
  line L1 (64.38, 43.235) -> (64.38, -43.235)
  line L2 (64.38, -43.235) -> (-64.38, -43.235)
  line L3 (-64.38, -43.235) -> (-64.38, 43.235)
  line L4 (-64.38, 43.235) -> (64.38, -43.235) construction
  line L5 (64.38, 43.235) -> (-64.38, -43.235) construction
  dimension "d18" = 128.76
  dimension "d19" = 86.47
  constraint perpendicular L0 L1
  constraint parallel L0 L2
  constraint parallel L1 L3
  constraint horizontal L0
  constraint coincident L4 origin
  constraint coincident L5 origin
  measures "d18" distance of L1.end L2.end
  measures "d19" distance of L0.end L1.end
extrude "Extrude2" cut sketch "Sketch2" against normal blind 4
sketch "Sketch3" plane through (0, 0, 3) normal (0, 0, 1) x (-1, 0, 0)
  line L0 (-64.38, -43.235) -> (-64.38, 43.235)
  line L1 (-64.38, 43.235) -> (64.38, 43.235)
  line L2 (64.38, 43.235) -> (64.38, -43.235)
  line L3 (64.38, -43.235) -> (-64.38, -43.235)
  line L4 (58.38, 57.37) -> (48.38, 57.37)
  line L5 (48.38, 57.37) -> (48.38, 47.37)
  line L6 (48.38, 47.37) -> (-48.38, 47.37)
  line L7 (-48.38, 47.37) -> (-48.38, 57.37)
  line L8 (-48.38, 57.37) -> (-58.38, 57.37)
  line L9 (-58.38, 57.37) -> (-58.38, 47.37)
  line L10 (-58.38, 47.37) -> (-68.38, 47.37)
  line L11 (-68.38, 47.37) -> (-68.38, -47.37)
  line L12 (-68.38, -47.37) -> (-58.38, -47.37)
  line L13 (-58.38, -47.37) -> (-58.38, -57.37)
  line L14 (-58.38, -57.37) -> (-48.38, -57.37)
  line L15 (-48.38, -57.37) -> (-48.38, -47.37)
  line L16 (-48.38, -47.37) -> (48.38, -47.37)
  line L17 (48.38, -47.37) -> (48.38, -57.37)
  line L18 (48.38, -57.37) -> (58.38, -57.37)
  line L19 (58.38, -57.37) -> (58.38, -47.37)
  line L20 (58.38, -47.37) -> (68.38, -47.37)
  line L21 (68.38, -47.37) -> (68.38, 47.37)
  line L22 (68.38, 47.37) -> (58.38, 47.37)
  line L23 (58.38, 47.37) -> (58.38, 57.37)
  circle A0 centre (53.38, -52.37) radius 3
  circle A1 centre (-53.38, -52.3704) radius 3
  circle A2 centre (-53.38, 52.3703) radius 3
  circle A3 centre (53.38, 52.37) radius 3
  dimension "d22" = 6
  dimension "d23" = 6
  dimension "d24" = 6
  dimension "d25" = 6
  measures "d22" diameter of A0
  measures "d23" diameter of A1
  measures "d24" diameter of A2
  measures "d25" diameter of A3
extrude "Extrude3" cut sketch "Sketch3" against normal blind 6 contours A0 | A1 | A2 | A3
fillet "Fillet1" radius 5 4 edges at (68.38, -47.37, 0) (68.38, 47.37, 0) (-68.38, -47.37, 0) (-68.38, 47.37, 0)
fillet "Fillet2" radius 2 4 edges at (64.38, 43.235, 1) (-64.38, 43.235, 1) (-64.38, -43.235, 1) (64.38, -43.235, 1)
fillet "Fillet3" radius 2 16 edges at (48.38, 47.37, 0) (48.38, 57.37, 0) (58.38, 57.37, 0) (-58.38, 47.37, 0) (-58.38, 57.37, 0) (-48.38, 57.37, 0) (-48.38, 47.37, 0) (58.38, 47.37, 0) (58.38, -47.37, 0) (58.38, -57.37, 0) (48.38, -57.37, 0) (-48.38, -47.37, 0) (-48.38, -57.37, 0) (48.38, -47.37, 0) (-58.38, -47.37, 0) (-58.38, -57.37, 0)

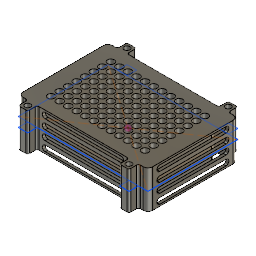
design "LED Spacer_96_v4_no_brim"
Autodesk Fusion 360 part; units mm, degrees
sketch "Sketch1" plane through (0, 0, 0) normal (0, 0, 1) x (1, 0, 0)
  line L0 (-68.38, 47.37) -> (68.38, 47.37)
  line L1 (68.38, 47.37) -> (68.38, -47.37)
  line L2 (68.38, -47.37) -> (-68.38, -47.37)
  line L3 (-68.38, -47.37) -> (-68.38, 47.37)
  line L4 (-68.38, 47.37) -> (68.38, -47.37) construction
  line L5 (68.38, 47.37) -> (-68.38, -47.37) construction
  line L6 (-58.38, 57.37) -> (-48.38, 57.37)
  line L7 (-48.38, 57.37) -> (-48.38, 47.37)
  line L8 (-48.38, 47.37) -> (-58.38, 47.37)
  line L9 (-58.38, 47.37) -> (-58.38, 57.37)
  line L10 (48.38, 57.37) -> (58.38, 57.37)
  line L11 (58.38, 57.37) -> (58.38, 47.37)
  line L12 (58.38, 47.37) -> (48.38, 47.37)
  line L13 (48.38, 47.37) -> (48.38, 57.37)
  line L14 (48.38, -47.37) -> (58.38, -47.37)
  line L15 (58.38, -47.37) -> (58.38, -57.37)
  line L16 (58.38, -57.37) -> (48.38, -57.37)
  line L17 (48.38, -57.37) -> (48.38, -47.37)
  line L18 (-58.38, -47.37) -> (-48.38, -47.37)
  line L19 (-48.38, -47.37) -> (-48.38, -57.37)
  line L20 (-48.38, -57.37) -> (-58.38, -57.37)
  line L21 (-58.38, -57.37) -> (-58.38, -47.37)
  point P0 (-53.88, -84.89)
  dimension "d1" = 136.76
  dimension "d2" = 94.74
  dimension "d3" = 10
  dimension "d4" = 10
  dimension "d5" = 10
  dimension "d6" = 10
  constraint perpendicular L0 L1
  constraint parallel L0 L2
  constraint parallel L1 L3
  constraint horizontal L0
  constraint horizontal L6
  constraint vertical L7
  constraint horizontal L8
  constraint vertical L9
  constraint coincident L0 L7.end
  constraint horizontal L10
  constraint vertical L11
  constraint horizontal L12
  constraint vertical L13
  constraint horizontal L14
  constraint vertical L15
  constraint horizontal L16
  constraint vertical L17
  constraint horizontal L18
  constraint vertical L19
  constraint horizontal L20
  constraint vertical L21
  measures "d1" distance of L1 L3
  measures "d2" distance of L0.start L2.end
  measures "d3" distance of L6.start L6.end
  measures "d4" distance of L6.start L8.end
  measures "d5" distance of L10.start L10.end
  measures "d6" distance of L10.start L12.end
extrude "Extrude26" add sketch "Sketch1" along normal blind 20 and the other way blind 20
ref_plane "WorkPlane26" through (0, 0, 20) normal (0, 0, 1) x (1, 0, 0)
sketch "Sketch25" plane through (0, 0, 20) normal (0, 0, 1) x (1, 0, 0)
  line L0 (49.5, -31.5) -> (-49.5, 31.5) construction
  line L1 (-49.5, -31.5) -> (49.5, 31.5) construction
  circle A0 centre (-49.5, -31.5) radius 3.575
  circle A1 centre (-40.5, -31.5) radius 3.575
  circle A2 centre (-31.5, -31.5) radius 3.575
  circle A3 centre (-22.5, -31.5) radius 3.575
  circle A4 centre (-13.5, -31.5) radius 3.575
  circle A5 centre (-4.5, -31.5) radius 3.575
  circle A6 centre (4.5, -31.5) radius 3.575
  circle A7 centre (13.5, -31.5) radius 3.575
  circle A8 centre (22.5, -31.5) radius 3.575
  circle A9 centre (31.5, -31.5) radius 3.575
  circle A10 centre (40.5, -31.5) radius 3.575
  circle A11 centre (49.5, -31.5) radius 3.575
  circle A12 centre (-49.5, -22.5) radius 3.575
  circle A13 centre (-40.5, -22.5) radius 3.575
  circle A14 centre (-31.5, -22.5) radius 3.575
  circle A15 centre (-22.5, -22.5) radius 3.575
  circle A16 centre (-13.5, -22.5) radius 3.575
  circle A17 centre (-4.5, -22.5) radius 3.575
  circle A18 centre (4.5, -22.5) radius 3.575
  circle A19 centre (13.5, -22.5) radius 3.575
  circle A20 centre (22.5, -22.5) radius 3.575
  circle A21 centre (31.5, -22.5) radius 3.575
  circle A22 centre (40.5, -22.5) radius 3.575
  circle A23 centre (49.5, -22.5) radius 3.575
  circle A24 centre (-49.5, -13.5) radius 3.575
  circle A25 centre (-40.5, -13.5) radius 3.575
  circle A26 centre (-31.5, -13.5) radius 3.575
  circle A27 centre (-22.5, -13.5) radius 3.575
  circle A28 centre (-13.5, -13.5) radius 3.575
  circle A29 centre (-4.5, -13.5) radius 3.575
  circle A30 centre (4.5, -13.5) radius 3.575
  circle A31 centre (13.5, -13.5) radius 3.575
  circle A32 centre (22.5, -13.5) radius 3.575
  circle A33 centre (31.5, -13.5) radius 3.575
  circle A34 centre (40.5, -13.5) radius 3.575
  circle A35 centre (49.5, -13.5) radius 3.575
  circle A36 centre (-49.5, -4.5) radius 3.575
  circle A37 centre (-40.5, -4.5) radius 3.575
  circle A38 centre (-31.5, -4.5) radius 3.575
  circle A39 centre (-22.5, -4.5) radius 3.575
  circle A40 centre (-13.5, -4.5) radius 3.575
  circle A41 centre (-4.5, -4.5) radius 3.575
  circle A42 centre (4.5, -4.5) radius 3.575
  circle A43 centre (13.5, -4.5) radius 3.575
  circle A44 centre (22.5, -4.5) radius 3.575
  circle A45 centre (31.5, -4.5) radius 3.575
  circle A46 centre (40.5, -4.5) radius 3.575
  circle A47 centre (49.5, -4.5) radius 3.575
  circle A48 centre (-49.5, 4.5) radius 3.575
  circle A49 centre (-40.5, 4.5) radius 3.575
  circle A50 centre (-31.5, 4.5) radius 3.575
  circle A51 centre (-22.5, 4.5) radius 3.575
  circle A52 centre (-13.5, 4.5) radius 3.575
  circle A53 centre (-4.5, 4.5) radius 3.575
  circle A54 centre (4.5, 4.5) radius 3.575
  circle A55 centre (13.5, 4.5) radius 3.575
  circle A56 centre (22.5, 4.5) radius 3.575
  circle A57 centre (31.5, 4.5) radius 3.575
  circle A58 centre (40.5, 4.5) radius 3.575
  circle A59 centre (49.5, 4.5) radius 3.575
  circle A60 centre (-49.5, 13.5) radius 3.575
  circle A61 centre (-40.5, 13.5) radius 3.575
  circle A62 centre (-31.5, 13.5) radius 3.575
  circle A63 centre (-22.5, 13.5) radius 3.575
  circle A64 centre (-13.5, 13.5) radius 3.575
  circle A65 centre (-4.5, 13.5) radius 3.575
  circle A66 centre (4.5, 13.5) radius 3.575
  circle A67 centre (13.5, 13.5) radius 3.575
  circle A68 centre (22.5, 13.5) radius 3.575
  circle A69 centre (31.5, 13.5) radius 3.575
  circle A70 centre (40.5, 13.5) radius 3.575
  circle A71 centre (49.5, 13.5) radius 3.575
  circle A72 centre (-49.5, 22.5) radius 3.575
  circle A73 centre (-40.5, 22.5) radius 3.575
  circle A74 centre (-31.5, 22.5) radius 3.575
  circle A75 centre (-22.5, 22.5) radius 3.575
  circle A76 centre (-13.5, 22.5) radius 3.575
  circle A77 centre (-4.5, 22.5) radius 3.575
  circle A78 centre (4.5, 22.5) radius 3.575
  circle A79 centre (13.5, 22.5) radius 3.575
  circle A80 centre (22.5, 22.5) radius 3.575
  circle A81 centre (31.5, 22.5) radius 3.575
  circle A82 centre (40.5, 22.5) radius 3.575
  circle A83 centre (49.5, 22.5) radius 3.575
  circle A84 centre (-49.5, 31.5) radius 3.575
  circle A85 centre (-40.5, 31.5) radius 3.575
  circle A86 centre (-31.5, 31.5) radius 3.575
  circle A87 centre (-22.5, 31.5) radius 3.575
  circle A88 centre (-13.5, 31.5) radius 3.575
  circle A89 centre (-4.5, 31.5) radius 3.575
  circle A90 centre (4.5, 31.5) radius 3.575
  circle A91 centre (13.5, 31.5) radius 3.575
  circle A92 centre (22.5, 31.5) radius 3.575
  circle A93 centre (31.5, 31.5) radius 3.575
  circle A94 centre (40.5, 31.5) radius 3.575
  circle A95 centre (49.5, 31.5) radius 3.575
  dimension "d242" = 99
  dimension "d243" = 63
  dimension "d244" = 7.15
  dimension "d247" = 99
  dimension "d248" = 63
  constraint coincident L0 origin
  constraint coincident L1 origin
  constraint coincident L1.start A0.centre
  measures "d242" distance of L0.end L1.end
  measures "d243" distance of L1.start L0.end
  measures "d244" diameter of A0
extrude "Extrude27" cut sketch "Sketch25" against normal blind 30
ref_plane "WorkPlane27" through (0, 0, -20) normal (0, 0, -1) x (-1, 0, 0)